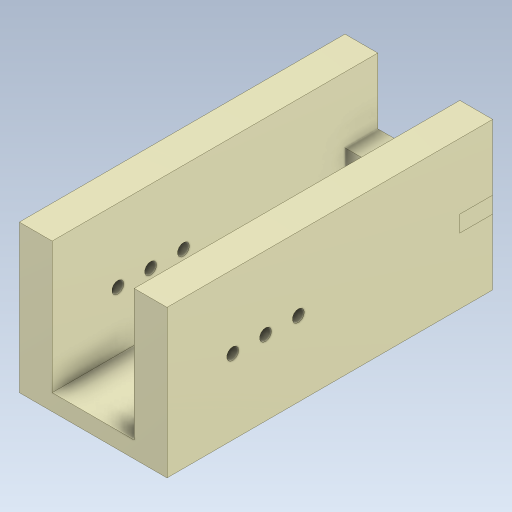
# Autodesk Inventor part: case
Saved by Autodesk Inventor 2024 (Build 280153000, 153)
## iProperties
Created: 2024-11-10
Part Number: case
Material: ABS Plastic
Document SubType Name: Modeling
Designer: Oscar
Density: 1.06 g/cm^3
Appearance: Smooth - Ash
Author: Oscar
Autodesk Inventor part; units mm, degrees
ref_plane "YZ Plane" through (0, 0, 0) normal (1, 0, 0) x (0, 1, 0)
ref_plane "XZ Plane" through (0, 0, 0) normal (0, 1, 0) x (-1, 0, 0)
ref_plane "XY Plane" through (0, 0, 0) normal (0, 0, 1) x (1, 0, 0)
sketch "Sketch1" plane through (0, 0, 0) normal (0, 1, 0) x (-1, 0, 0)
  line L0 (0, 0) -> (57.15, 0)
  line L1 (57.15, 0) -> (57.15, -126)
  line L2 (57.15, -126) -> (0, -126)
  line L3 (0, -126) -> (0, 0)
  dimension "d0" = 57.15
  dimension "d1" = 126
  constraints: 8 end point, 2 parallel, 1 horizontal, 1 perpendicular
  measures "d0" distance between parallel lines of L1 L3
  measures "d1" distance between parallel lines of L2 L0
extrude "Extrusion1" add sketch "Sketch1" along normal blind 6.35
sketch "Sketch2" plane through (0, 6.35, 0) normal (0, 1, 0) x (1, 0, 0)
  line L0 (-57.15, 0) -> (0, 0) projected
  line L1 (0, 126) -> (-57.15, 126) projected
  line L2 (-57.15, 0) -> (-44.45, 0)
  line L3 (-44.45, 0) -> (-44.45, 126)
  line L4 (-44.45, 126) -> (-57.15, 126)
  line L5 (-57.15, 126) -> (-57.15, 0)
  line L6 (0, 0) -> (-12.7, 0)
  line L7 (-12.7, 0) -> (-12.7, 126)
  line L8 (-12.7, 126) -> (0, 126)
  line L9 (0, 126) -> (0, 0)
  dimension "d4" = 12.7
  dimension "d5" = 12.7
  constraints: 16 end point, 4 parallel, 2 horizontal, 2 perpendicular, 2 point on line
  measures "d4" distance of L4.end L3.end
  measures "d5" distance of L7.end L8.end
extrude "Extrusion2" add sketch "Sketch2" along normal blind 50.8 contours L5 L1 L3 L0 | L7 L1 L9 L0
sketch "Sketch3" plane through (-57.15, 0, -126) normal (-1, 0, 0) x (0, 0, 1)
  line L0 (0, 6.35) -> (126, 6.35) construction
  line L1 (0, 0) -> (126, 0) construction
  line L2 (126, 0) -> (126, 6.35) construction
  line L3 (126, 6.35) -> (0, 6.35) construction
  line L4 (0, 6.35) -> (0, 0) construction
  line L5 (-0.0082, 18.796) -> (126.0082, 18.796) construction
  circle A0 centre (100.6, 28.956) radius 10.16 construction
  circle A1 centre (87.9, 28.956) radius 2.3114
  circle A2 centre (75.2, 28.956) radius 2.3114
  circle A3 centre (100.6, 28.956) radius 2.3114
  line L6 (126, 0) -> (126, 57.15) projected
  dimension "d8" = 12.446
  dimension "d9" = 20.32
  dimension "d10" = 4.6228
  dimension "d11" = 12.7
  dimension "d12" = 12.7
  dimension "d14" = 25.4
  constraints: 10 end point, 4 centre point, 2 equal radius, 2 horizontal, 2 horizontal alignment, 2 parallel, 1 coincident, 1 perpendicular, 1 tangent
  measures "d8" distance between parallel lines of L5 L0
  measures "d9" diameter of A0
  measures "d10" diameter of A1
  measures "d11" distance of A1.centre A2.centre
  measures "d12" distance of A0.centre A1.centre
  measures "d14" distance from line of L6 A0.centre
extrude "Extrusion3" cut sketch "Sketch3" against normal through all
sketch "Sketch4" plane through (-57.15, 0, -126) normal (-1, 0, 0) x (0, 0, 1)
  line L0 (0, 0) -> (126, 0) projected
  line L1 (0, 6.35) -> (126, 6.35) projected
  line L2 (0, 0) -> (126, 0)
  line L3 (126, 0) -> (126, 6.35)
  line L4 (126, 6.35) -> (0, 6.35)
  line L5 (0, 6.35) -> (0, 0)
  line L6 (0, 0) -> (0, 57.15) projected
  line L7 (0, 18.796) -> (126, 18.796) construction
  line L8 (0, 31.75) -> (12.7, 31.75)
  line L9 (12.7, 31.75) -> (12.7, 25.4)
  line L10 (12.7, 25.4) -> (0, 25.4)
  line L11 (0, 25.4) -> (0, 31.75)
  point P0 (0, 25.4)
  dimension "d17" = 12.446
  dimension "d18" = 12.7
  dimension "d19" = 6.35
  dimension "d21" = 19.05
  constraints: 18 end point, 4 parallel, 3 horizontal, 2 perpendicular, 2 point on line
  measures "d17" distance between parallel lines of L7 L1
  measures "d18" distance of L9.end L10.end
  measures "d19" distance of L8.end L9.end
  measures "d21" distance between parallel lines of L10 L1
extrude "Extrusion4" add sketch "Sketch4" against normal through all separate body contours L6 L8 L9 L10
body "Solid1"
body "Solid2"
